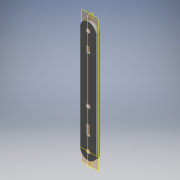
# Autodesk Inventor part: Part5
Saved by Autodesk Inventor 2019.2 (Build 232265000, 265)
## iProperties
Part Number: Part5
Material: Generic
Document SubType Name: Modeling
Designer: richard.girt
Mass: 2.8113 g
Surface Area: 27.6263 cm^2
Volume: 2.8113 cm^3
Density: 1 g/cm^3
Appearance: Default
Author: richard.girt
Autodesk Inventor part; units mm, degrees
ref_plane "YZ Plane" through (0, 0, 0) normal (1, 0, 0) x (0, 1, 0)
ref_plane "XZ Plane" through (0, 0, 0) normal (0, 1, 0) x (-1, 0, 0)
ref_plane "XY Plane" through (0, 0, 0) normal (0, 0, 1) x (1, 0, 0)
sketch "Sketch1" plane through (0, 0, 0) normal (0, 0, 1) x (1, 0, 0)
  circle A0 centre (0, 0) radius 6
  line L0 (0, 0) -> (0, 80) construction
  line L1 (6, 0) -> (6, 80)
  line L2 (-6, 80) -> (-6, 0)
  arc A1 (-6, 0) -> (6, 0) centre (0, 0) ccw
  arc A2 (6, 80) -> (-6, 80) centre (0, 80) ccw
  point P0 (0, 40)
  dimension "d0" = 12
  dimension "d1" = 12
  dimension "d2" = 80
  constraints: 8 end point, 5 tangent, 4 point on circle, 3 centre point, 2 coincident, 1 midpoint, 1 parallel, 1 vertical
  measures "d0" diameter of A0
  measures "d1" distance between parallel lines of L1 L2
  measures "d2" distance of point (0, 0) L0.end
extrude "Extrusion1" add sketch "Sketch1" along normal mid plane 2.8
sketch "Sketch2" plane through (0, 0, 1.4) normal (0, 0, 1) x (1, 0, 0)
  arc A0 (6, 80) -> (-6, 80) centre (0, 80) ccw construction
  arc A1 (-6, 0) -> (6, 0) centre (0, 0) ccw construction
  circle A2 centre (0, 0) radius 1.75
  circle A3 centre (0, 80) radius 1.75
  line L0 (-1.5, 64.9) -> (1.5, 64.9)
  line L1 (1.5, 64.9) -> (1.5, 70.1)
  line L2 (1.5, 70.1) -> (-1.5, 70.1)
  line L3 (-1.5, 70.1) -> (-1.5, 64.9)
  circle A4 centre (0, 30) radius 1.75
  line L4 (-1.5, 9.9) -> (1.5, 9.9)
  line L5 (1.5, 9.9) -> (1.5, 18.1)
  line L6 (1.5, 18.1) -> (-1.5, 18.1)
  line L7 (-1.5, 18.1) -> (-1.5, 9.9)
  point P0 (0, 9.9)
  point P1 (0, 64.9)
  point P2 (1.5, 14)
  point P3 (1.5, 67.5)
  dimension "d8" = 3.5
  dimension "d9" = 3.5
  dimension "d12" = 3
  dimension "d13" = 8.2
  dimension "d16" = 5.2
  dimension "d18" = 14
  dimension "d19" = 30
  dimension "d20" = 12.5
  constraints: 16 end point, 5 parallel, 4 midpoint, 3 centre point, 3 vertical alignment, 2 coincident, 2 horizontal, 2 perpendicular, 1 equal radius
  measures "d8" diameter of A3
  measures "d9" diameter of A2
  measures "d12" distance of L5.end L6.end
  measures "d13" distance of L4.end L5.end
  measures "d16" distance of L0.end L1.end
  measures "d18" vertical distance of point (1.5, 14) A1.centre
  measures "d19" distance of A4.centre A1.centre
  measures "d20" vertical distance of point (1.5, 67.5) A0.centre
extrude "Extrusion2" cut sketch "Sketch2" against normal through all
body "Solid1"
